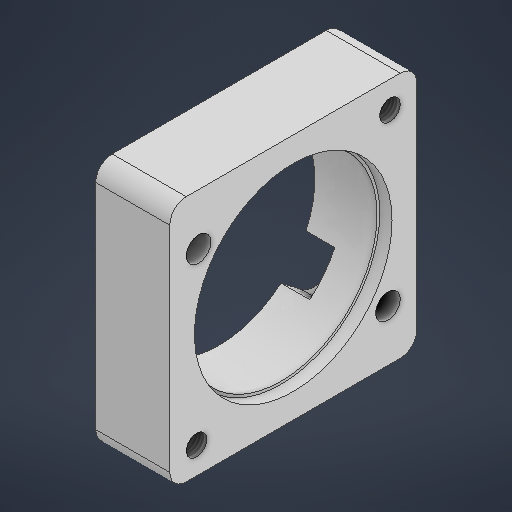
# Autodesk Inventor part: Mounting Bracket
Saved by Autodesk Inventor 2027 (Build 310192000, 192)
## iProperties
Created: 2026-05-27
Part Number: Mounting Bracket
Material: Generic
Document SubType Name: Modeling
Designer: ratik
Density: 1 g/cm^3
Appearance: Default
Author: ratik
Autodesk Inventor part; units mm, degrees
ref_plane "YZ Plane" through (0, 0, 0) normal (1, 0, 0) x (0, 1, 0)
ref_plane "XZ Plane" through (0, 0, 0) normal (0, 1, 0) x (-1, 0, 0)
ref_plane "XY Plane" through (0, 0, 0) normal (0, 0, 1) x (1, 0, 0)
sketch "Sketch1" plane through (0, 0, 0) normal (1, 0, 0) x (0, 1, 0)
  line L0 (30, 30) -> (-30, 30)
  line L1 (-30, 30) -> (-30, -30)
  line L2 (-30, -30) -> (30, -30)
  line L3 (30, -30) -> (30, 30)
  line L4 (30, 30) -> (-30, -30) construction
  line L5 (-30, 30) -> (30, -30) construction
  point P0 (0, 0)
  dimension "d0" = 60
  dimension "d1" = 60
  constraints: 12 end point, 2 midpoint, 2 parallel, 1 horizontal, 1 perpendicular
  measures "d0" distance of L2.end L0.start
  measures "d1" distance of L0.start L0.end
extrude "Extrusion1" add sketch "Sketch1" along normal blind 18
fillet "Fillet1" radius 4 4 edges at (9, 30, 30) (9, 30, -30) (9, -30, 30) (9, -30, -30)
sketch "Sketch2" plane through (0, 0, 0) normal (-1, 0, 0) x (0, 0, 1)
  circle A0 centre (0, 0) radius 24.15
  dimension "d5" = 48.3
  constraints: 1 centre point, 1 coincident
  measures "d5" diameter of A0
extrude "Extrusion2" add sketch "Sketch2" along normal blind 0.1
sketch "Sketch3" plane through (-0.1, 0, 0) normal (-1, 0, 0) x (0, 0, 1)
  circle A0 centre (0, 0) radius 23.35
  dimension "d8" = 46.7
  constraints: 1 centre point, 1 coincident
  measures "d8" diameter of A0
extrude "Extrusion3" cut sketch "Sketch3" against normal through all
sketch "Sketch4" plane through (18, 0, 0) normal (1, 0, 0) x (0, 0, -1)
  circle A0 centre (0, 0) radius 24
  dimension "d11" = 48
  constraints: 1 centre point, 1 coincident
  measures "d11" diameter of A0
extrude "Extrusion4" cut sketch "Sketch4" against normal blind 3
sketch "Sketch5" plane through (0, 0, 0) normal (-1, 0, 0) x (0, 0, 1)
  point P0 (0, 0)
sketch "Sketch6" plane through (0, 0, 0) normal (-1, 0, 0) x (0, 0, 1)
  circle A0 centre (23, 17.5) radius 3
  line L0 (30, 26) -> (30, -26) projected
  line L1 (-26, 30) -> (26, 30) projected
  circle A1 centre (-23, -17.5) radius 3
  line L2 (-30, -26) -> (-30, 26) projected
  line L3 (26, -30) -> (-26, -30) projected
  circle A2 centre (-23.5, 23.5) radius 2.5
  circle A3 centre (23.5, -23.5) radius 2.5
  point P0 (0, 0)
  dimension "d15" = 7
  dimension "d16" = 12.5
  dimension "d17" = 6
  dimension "d18" = 6
  dimension "d19" = 7
  dimension "d20" = 12.5
  dimension "d21" = 23.5
  dimension "d22" = 23.5
  dimension "d23" = 23.5
  dimension "d24" = 23.5
  dimension "d25" = 5
  dimension "d26" = 5
  constraints: 4 centre point
  measures "d15" distance from line of L0 A0.centre
  measures "d16" distance from line of L1 A0.centre
  measures "d17" diameter of A0
  measures "d18" diameter of A1
  measures "d19" distance from line of L2 A1.centre
  measures "d20" distance from line of L3 A1.centre
  measures "d21" horizontal distance of A2.centre point (0, 0)
  measures "d22" horizontal distance of point (0, 0) A2.centre
  measures "d23" horizontal distance of point (0, 0) A3.centre
  measures "d24" horizontal distance of point (0, 0) A3.centre
  measures "d25" diameter of A2
  measures "d26" diameter of A3
extrude "Extrusion5" cut sketch "Sketch6" against normal through all
sketch "Sketch7" plane through (-0.1, 0, 0) normal (-1, 0, 0) x (0, 0, 1)
  circle A0 centre (-23, -17.5) radius 3 projected
  circle A1 centre (23, 17.5) radius 3 projected
  line L0 (-23, -17.5) -> (23, 17.5) construction
  line L1 (-19.9724, -21.4791) -> (26.0276, 13.5209)
  line L2 (19.9724, 21.4791) -> (-26.0276, -13.5209)
  arc A2 (-26.0276, -13.5209) -> (-19.9724, -21.4791) centre (-23, -17.5) ccw
  arc A3 (26.0276, 13.5209) -> (19.9724, 21.4791) centre (23, 17.5) ccw
  point P0 (0, 0)
  point P1 (0, 0)
  dimension "d29" = 10
  constraints: 8 end point, 4 point on circle, 4 tangent, 2 centre point, 1 midpoint, 1 parallel
  measures "d29" diameter of A3
extrude "Extrusion6" cut sketch "Sketch7" against normal blind 7
thread "Thread1" size "M5x0.8" class "6H" standard "ANSI Metric M Profile" full length
thread "Thread2" size "M5x0.8" class "6H" standard "ANSI Metric M Profile" full length
body "Solid1"
